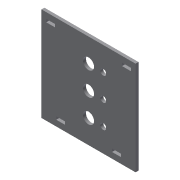
# Autodesk Inventor part: fishpaper
Saved by Autodesk Inventor 2022 (Build 260148000, 148)
## iProperties
Shininess: 64.0
Length Units: 11272
Angle Units: 11279
Time Units: 11290
Mass Units: 11286
Length Display Precision: 3
Angle Display Precision: 2
Created: 2002-05-01
Part Number: fishpaper
Document SubType Name: Modeling
Designer: Administrator
Density: 1 g/cm^3
Material: Generic
Appearance: Default
Density: 0.0
Volumn: 0.0
Area: 0.0
PropertySet Name: Model Information
Control State: 0
Master: False
Checked Out: False
Author: Administrator
Autodesk Inventor part; units mm, degrees
ref_plane "YZ Plane" through (0, 0, 0) normal (1, 0, 0) x (0, 1, 0)
ref_plane "XZ Plane" through (0, 0, 0) normal (0, 1, 0) x (-1, 0, 0)
ref_plane "XY Plane" through (0, 0, 0) normal (0, 0, 1) x (1, 0, 0)
sketch "Sketch1" plane through (0, 0, 0) normal (0, 0, 1) x (1, 0, 0)
  line L0 (-18.6192, 22.6484) -> (22.0208, 22.6484)
  line L1 (22.0208, 22.6484) -> (22.0208, -17.9916)
  line L2 (22.0208, -17.9916) -> (-18.6192, -17.9916)
  line L3 (-18.6192, -17.9916) -> (-18.6192, 22.6484)
  dimension "d0" = 40.64
  dimension "d1" = 40.64
  constraints: 8 end point, 2 parallel, 1 horizontal, 1 perpendicular
  measures "d0" distance of L2.end L0.start
  measures "d1" distance of L0.start L0.end
extrude "Extrusion1" add sketch "Sketch1" along normal blind 1.27
sketch "Sketch2" plane through (0, 0, 1.27) normal (0, 0, 1) x (1, 0, 0)
  line L0 (-18.6192, 22.6484) -> (22.0208, 22.6484) projected
  line L1 (-18.6192, -17.9916) -> (-18.6192, 22.6484) projected
  line L2 (-16.5872, 20.1084) -> (-12.7772, 20.1084)
  line L3 (-12.7772, 20.1084) -> (-12.7772, 18.8384)
  line L4 (-12.7772, 18.8384) -> (-16.5872, 18.8384)
  line L5 (-16.5872, 18.8384) -> (-16.5872, 20.1084)
  dimension "d4" = 2.54
  dimension "d5" = 1.27
  dimension "d6" = 2.032
  dimension "d7" = 3.81
  constraints: 8 end point, 2 parallel, 1 horizontal, 1 perpendicular
  measures "d4" distance between parallel lines of L0 L2
  measures "d5" distance of L4.end L2.start
  measures "d6" distance from line of L2.start L1
  measures "d7" distance of L2.start L2.end
extrude "Extrusion2" cut sketch "Sketch2" against normal through all
pattern_linear "Rectangular Pattern1" count 2 spacing 32.766 along (1, 0, 0) of "Extrusion2"
sketch "Sketch3" plane through (0, 0, 1.27) normal (0, 0, 1) x (1, 0, 0)
  line L0 (22.0208, 22.6484) -> (22.0208, -17.9916) projected
  line L1 (-18.6192, 22.6484) -> (22.0208, 22.6484) projected
  line L2 (-18.6192, -17.9916) -> (-18.6192, 22.6484) projected
  circle A0 centre (1.7008, 12.4884) radius 2.3876
  circle A1 centre (8.0508, 12.4884) radius 1.27
  circle A2 centre (1.7008, 12.4884) radius 20.32 construction
  dimension "d16" = 2.54
  dimension "d17" = 4.7752
  dimension "d18" = 6.35
  dimension "d19" = 10.16
  constraints: 3 centre point, 2 tangent, 1 coincident, 1 horizontal alignment
  measures "d16" diameter of A1
  measures "d17" diameter of A0
  measures "d18" distance of A1.centre A0.centre
  measures "d19" distance from line of L1 A0.centre
extrude "Extrusion3" cut sketch "Sketch3" against normal through all
pattern_linear "Rectangular Pattern2" count 3 spacing 10.16 along (0, -1, 0) of "Extrusion3"
sketch "Sketch4" plane through (0, 0, 1.27) normal (0, 0, 1) x (1, 0, 0)
  line L0 (-18.6192, -17.9916) -> (-18.6192, 22.6484) projected
  line L1 (22.0208, -17.9916) -> (-18.6192, -17.9916) projected
  line L2 (-12.2692, -15.4516) -> (-8.4592, -15.4516)
  line L3 (-8.4592, -15.4516) -> (-8.4592, -14.1816)
  line L4 (-8.4592, -14.1816) -> (-12.2692, -14.1816)
  line L5 (-12.2692, -14.1816) -> (-12.2692, -15.4516)
  dimension "d25" = 3.81
  dimension "d26" = 1.27
  dimension "d27" = 2.54
  dimension "d28" = 6.35
  constraints: 8 end point, 2 parallel, 1 horizontal, 1 perpendicular
  measures "d25" distance of L2.start L2.end
  measures "d26" distance of L4.end L2.start
  measures "d27" distance from line of L2.start L1
  measures "d28" distance from line of L2.start L0
extrude "Extrusion4" cut sketch "Sketch4" against normal through all
pattern_linear "Rectangular Pattern3" count 2 spacing 24.13 along (1, 0, 0) of "Extrusion4"
body "Solid1"
